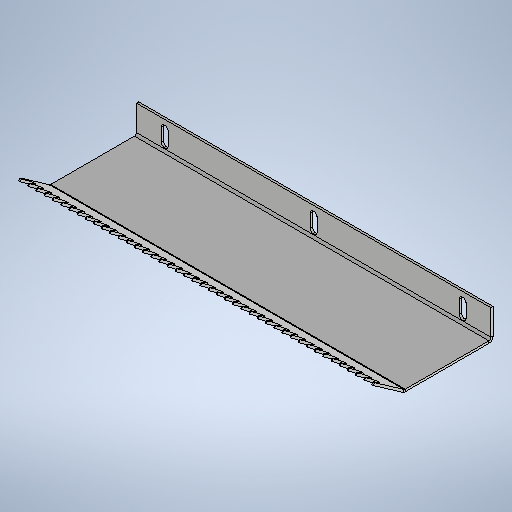
# Autodesk Inventor part: TRM 018 clipper
Saved by Autodesk Inventor 2025.1 (Build 291241020, 241B)
## iProperties
Created: 2024-08-07
Part Number: TRM 018 clipper
Material: AISI 304
Document SubType Name: Sheet Metal
Designer: pokla
Density: 8.02768 g/cm^3
Sheet Metal Rule: AISI304 2mm Die16
Sheet Metal Width: 203.753 mm
Sheet Metal Length: 476.000 mm
Sheet Metal Area: 96986.631 mm^2
Appearance: Default
Stock Number: ТРМ 018 отсекатель
Flat Pattern Width: 20.3753 cm
Flat Pattern Length: 47.6 cm
Flat Pattern Area: 969.866 cm^2
Author: pokla
Autodesk Inventor part; units mm, degrees
ref_plane "YZ Plane" through (0, 0, 0) normal (1, 0, 0) x (0, 1, 0)
ref_plane "XZ Plane" through (0, 0, 0) normal (0, 1, 0) x (-1, 0, 0)
ref_plane "XY Plane" through (0, 0, 0) normal (0, 0, 1) x (1, 0, 0)
sketch "Sketch1" plane through (0, 0, 0) normal (0, 0, 1) x (1, 0, 0)
  line L0 (-238, -60) -> (238, -60)
  line L1 (238, -60) -> (238, 60)
  line L2 (238, 60) -> (-238, 60)
  line L3 (-238, 60) -> (-238, -60)
  line L4 (-238, -60) -> (238, 60) construction
  line L5 (238, -60) -> (-238, 60) construction
  point P0 (0, 0)
  dimension "d0" = 476
  dimension "d1" = 120
  measures "d0" distance of L2.end L1.end
  measures "d1" distance of L1.end L0.end
extrude "Plate1" add sketch "Sketch1" along normal blind 3
sketch "Sketch6" plane through (0, 0, 3) normal (0, 0, 1) x (1, 0, 0)
  line L0 (238, -60) -> (-238, -60) projected
  line L1 (238, 60) -> (238, -60) projected
  line L2 (-238, 60) -> (238, 60) projected
  line L3 (-238, -60) -> (-238, 60) projected
  line L4 (-1.5, -50) -> (1.5, -50)
  line L5 (1.5, -50) -> (5.1397, -60)
  line L6 (-1.5, -50) -> (-5.1397, -60)
  point P0 (0, 0)
  point P1 (0, -50)
  point P2 (0, -60)
  dimension "d33" = 10
  dimension "d34" = 40
  dimension "d35" = 3
  constraints: 6 end point, 2 midpoint, 2 point on line, 1 equal length, 1 horizontal, 1 vertical alignment
  measures "d33" distance between parallel lines of L0 L4
  measures "d34" angle of L5 L6
  measures "d35" distance of L4.start L4.end
cut "Cut1" [suppressed]
pattern_linear "Rectangular Pattern1" [suppressed]
sketch "Sketch7" plane through (-238, 57, 0) normal (0, 1, 0) x (-1, 0, 0)
  line L0 (-476, 0) -> (0, 0)
  line L1 (0, 0) -> (0, 40)
  line L2 (0, 40) -> (-476, 40)
  line L3 (-476, 40) -> (-476, 0)
  constraints: 6 end point, 1 horizontal, 1 perpendicular, 1 vertical
edge flange "Flange3" height 40 angle 90 thickness 3 bend radius 2.75 thickness toward (0, 1, 0) relief round relief width 3 relief depth 1.5 edges at (0, 60, 3) wall of the first edge with corners at (238, 57, 0) (-238, 57, 0) (-238, 57, 40) (238, 57, 40)
bend "Bend3"
corner "Corner3"
sketch "Sketch8" plane through (-238, 60, 40) normal (0, 1, 0) x (1, 0, 0)
  line L0 (238, 29) -> (238, 11) construction
  line L1 (233.5, 29) -> (233.5, 11)
  line L2 (242.5, 11) -> (242.5, 29)
  arc A0 (242.5, 29) -> (233.5, 29) centre (238, 29) ccw
  arc A1 (233.5, 11) -> (242.5, 11) centre (238, 11) ccw
  point P0 (238, 40)
  point P1 (238, 20)
  dimension "d51" = 9
  dimension "d52" = 11
  dimension "d53" = 18
  constraints: 8 end point, 4 point on circle, 4 tangent, 2 centre point, 1 midpoint, 1 parallel, 1 vertical, 1 vertical alignment
  measures "d51" diameter of A1
  measures "d52" distance of point (238, 40) L0.start
  measures "d53" distance of L0.start L0.end
extrude "Cut2" cut sketch "Sketch8" against normal blind 3
pattern_linear "Rectangular Pattern2" count 3 spacing 200 along (-1, 0, 0) of "Cut2" first direction both ways yes
sketch "Sketch9" plane through (238, -58.2793, 2.4575) normal (0, -0.5735764, -0.819152) x (1, 0, 0)
  line L0 (-476, 0) -> (0, 0)
  line L1 (0, 0) -> (0, 50)
  line L2 (0, 50) -> (-476, 50)
  line L3 (-476, 50) -> (-476, 0)
  constraints: 6 end point, 1 horizontal, 1 perpendicular, 1 vertical
edge flange "Flange4" height 50 angle 35 thickness 3 bend radius 2.75 thickness toward (0, -0.5735764, -0.819152) relief round relief width 3 relief depth 1.5 edges at (0, -60, 3) wall of the first edge with corners at (-238, -58.2793, 2.4575) (238, -58.2793, 2.4575) (238, -99.2369, 31.1363) (-238, -99.2369, 31.1363)
bend "Bend4"
corner "Corner4"
sketch "Sketch10" plane through (238, -100.9576, 28.6788) normal (0, -0.5735764, -0.819152) x (-1, 0, 0)
  line L0 (476, 48.187) -> (0, 48.187) projected
  line L1 (0, 0) -> (0, 48.187) projected
  line L2 (476, 0) -> (0, 0) projected
  line L3 (476, 48.187) -> (476, 0) projected
  line L4 (243, 0) -> (239.5, 15)
  line L5 (239.5, 15) -> (236.5, 15)
  line L6 (236.5, 15) -> (233, 0)
  line L7 (476, 0) -> (0, 0) projected
  point P0 (238, 99.1491)
  point P1 (238, 15)
  point P2 (238, 48.187)
  dimension "d72" = 3
  dimension "d73" = 15
  dimension "d79" = 10
  constraints: 6 end point, 2 midpoint, 2 point on line, 1 equal length, 1 horizontal, 1 vertical alignment
  measures "d72" distance of L4.end L5.end
  measures "d73" distance between parallel lines of L5 L2
  measures "d79" distance of L4.start L6.end
extrude "Cut3" cut sketch "Sketch10" against normal blind 3 contours L2 L6 L5 L4
pattern_linear "Rectangular Pattern3" count 43 spacing 11 along (-1, 0, 0) of "Cut3" first direction both ways yes
equation "\"d36\" = Thickness"
equation "\"d54\" = Thickness"
equation "\"d74\" = Thickness"
equation "\"d2\" = Thickness"
equation "\"d41\" = BendReliefWidth"
equation "\"d42\" = BendReliefDepth"
equation "\"d43\" = MinimumRemnant"
equation "\"d44\" = TransitionRadius"
equation "\"d47\" = BendRadius"
equation "\"d48\" = CornerReliefSize"
equation "\"d49\" = GapSize"
equation "\"d50\" = JacobiRadiusSize"
equation "\"d59\" = BendReliefWidth"
equation "\"d60\" = BendReliefDepth"
equation "\"d61\" = MinimumRemnant"
equation "\"d62\" = TransitionRadius"
equation "\"d65\" = BendRadius"
equation "\"d66\" = CornerReliefSize"
equation "\"d67\" = GapSize"
equation "\"d68\" = JacobiRadiusSize"
equation "\"BendReliefWidth\" = Thickness"
equation "\"BendReliefDepth\" = 0.5 * Thickness"
equation "\"CornerReliefSize\" = 4 * Thickness"
equation "\"MinimumRemnant\" = 2 * Thickness"
equation "\"TransitionRadius\" = BendRadius"
equation "\"JacobiRadiusSize\" = BendRadius"
equation "\"GapSize\" = Thickness"
equation "\"Thickness\" = 3"
equation "\"BendRadius\" = 2.75"
body "Solid1"
